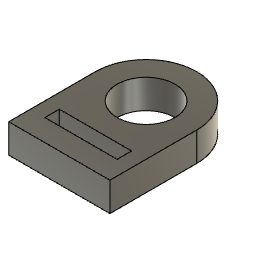
exercise1 (Autodesk Fusion 360 design; units mm, degrees)
Autodesk Fusion 360 part; units mm, degrees
sketch "Sketch1" plane through (0, 0, 0) normal (0, 0, 1) x (1, 0, 0)
  line L0 (0, 0) -> (70, 0)
  line L1 (70, 0) -> (70, 60)
  line L2 (0, 60) -> (0, 0)
  circle A0 centre (35, 60) radius 20
  line L3 (10, 25) -> (60, 25)
  line L4 (60, 25) -> (60, 15)
  line L5 (60, 15) -> (10, 15)
  line L6 (10, 15) -> (10, 25)
  arc A1 (70, 60) -> (0, 60) centre (35, 60) ccw
  dimension "d1" = 70
  dimension "d2" = 60
  dimension "d3" = 40
  dimension "d4" = 10
  dimension "d5" = 15
  dimension "d6" = 10
  dimension "d7" = 50
  constraint coincident L0.start L2.end
  constraint horizontal L0
  constraint vertical L1
  constraint vertical L2
  constraint tangent L1 A1
  constraint concentric A0 A1
  constraint horizontal L3
  constraint vertical L4
  constraint horizontal L5
  constraint vertical L6
  constraint tangent L2 A1
  constraint tangent L3 A1
  measures "d1" distance of L0.start L0.end
  measures "d2" distance of L0.end L1.end
  measures "d3" diameter of A0
  measures "d4" distance of L2 L6
  measures "d5" distance of L0 L5
  measures "d6" distance of L3.end L4.end
  measures "d7" distance of L4.end L5.end
extrude "Extrude1" add sketch "Sketch1" along normal blind 20
